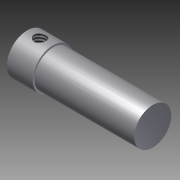
# Autodesk Inventor part: 13_1087_027
Saved by Autodesk Inventor 2014 (Build 180170000, 170)
## iProperties
Created: 2013-09-17
Part Number: 13_1087_027
Material: Allgemein
Document SubType Name: Modeling
Designer: vogel
Density: 1 g/cm^3
Appearance: Vorgabe
Author: vogel
Autodesk Inventor part; units mm, degrees
note: some values were not read from the file. Chosen so that the rebuilt part matches the saved one: direction of "Bohrung2".
ref_plane "YZ Plane" through (0, 0, 0) normal (1, 0, 0) x (0, 1, 0)
ref_plane "XZ Plane" through (0, 0, 0) normal (0, 1, 0) x (-1, 0, 0)
sketch "Skizze1" plane through (0, 0, 0) normal (0, 0, 1) x (1, 0, 0)
  line L0 (-3.4, 0) -> (20.4, 0) projected
  line L1 (0, -0.55) -> (0, 3.3) projected
  line L2 (0, 2.75) -> (3.5, 2.75)
  line L3 (3.5, 2.75) -> (3.5, 2.5)
  line L4 (3.5, 2.5) -> (17, 2.5)
  line L5 (17, 2.5) -> (17, 0)
  line L6 (17, 0) -> (0, 0)
  line L7 (0, 0) -> (0, 2.75)
  dimension "d0" = 5.5
  dimension "d1" = 5
  dimension "d2" = 3.5
  dimension "d3" = 17
  constraints: 12 end point, 3 perpendicular, 2 parallel, 2 point on line, 1 collinear
  measures "d0" diameter of L2 L0
  measures "d1" diameter of L4 L0
  measures "d2" distance of L2.start L2.end
  measures "d3" distance between parallel lines of L5 L1
revolve "Umdrehung1" add sketch "Skizze1" angle 360 about axis through (-10, 0, 0) along (1, 0, 0)
hole "Bohrung1" at (0, 0, 0) direction (1, 0, 0) diameter 3 depth 6 tip angle 118
ref_plane "Arbeitsebene1" through (1.75, 0, 2.75) normal (0, 0, 1) x (1, 0, 0)
sketch "Skizze2" plane through (1.75, 0, 2.75) normal (0, 0, 1) x (1, 0, 0)
  line L0 (-5.15, 0) -> (18.65, 0) projected
  line L1 (-1.75, -3.85) -> (-1.75, 3.85) projected
  point P0 (-1.75, 0)
  point P1 (0, 0)
  dimension "d14" = 1.75
  constraints: 1 point on line
  measures "d14" distance from line of point (0, 0) L1
hole "Bohrung2" at (1.75, 0, 2.75) direction (0, 0, -1) diameter 1.567 end up to surface thread size "M2x0.4" class "6H" standard "ISO Metric profile"
